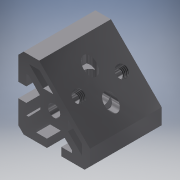
# Autodesk Inventor part: 21-035
Saved by Autodesk Inventor 2018 (Build 220105000, 105)
## iProperties
Created: 2004-10-14
Part Number: 21-035
Material: Aluminum-6061
Document SubType Name: Modeling
Designer: Autodesk, Inc.
Manufacturer: Standard
Standards Organization: Custom
Description: CORNER ELEMENT 1, 40
Catalog Web Link: http://www.parker.com/ead/cm1.asp?cmid=809
Vendor: PARKER IPS
Mass: 78.2567 g
Surface Area: 142.922 cm^2
Volume: 28.877 cm^3
Density: 2.71 g/cm^3
Appearance: Metal-AL-6061 (Polished)
CAGE: 1LJX3
Dept. ID: Product Design
Description #2: ---
Finish #1: ---
Finish #2: ---
Material ID: ---
Project Number: ---
Author: Autodesk, Inc.
Autodesk Inventor part; units mm, degrees
note: some values were not read from the file. Chosen so that the rebuilt part matches the saved one: direction of "Mounting Hole".
ref_plane "YZ Plane" through (0, 0, 0) normal (1, 0, 0) x (0, 1, 0)
ref_plane "XZ Plane" through (0, 0, 0) normal (0, 1, 0) x (-1, 0, 0)
sketch "Sketch1" plane through (0, 0, 0) normal (0, 0, 1) x (1, 0, 0)
  circle A0 centre (0, 0) radius 3.4
  line L0 (-8.3327, 20) -> (20, -8.3327)
  line L1 (20, -8.3327) -> (20, -17)
  line L2 (20, -17) -> (17, -20)
  line L3 (17, -20) -> (4, -20)
  line L4 (4, -20) -> (4, -15.5)
  line L5 (4, -15.5) -> (10, -15.5)
  line L6 (10, -15.5) -> (10, -14.177)
  line L7 (10, -14.177) -> (3.3741, -7.75)
  line L8 (3.3741, -7.75) -> (-3.3741, -7.75)
  line L9 (-3.3741, -7.75) -> (-10, -14.177)
  line L10 (-10, -14.177) -> (-10, -15.5)
  line L11 (-10, -15.5) -> (-4, -15.5)
  line L12 (-4, -15.5) -> (-4, -20)
  line L13 (-4, -20) -> (-17, -20)
  line L14 (-17, -20) -> (-20, -17)
  line L15 (-20, -17) -> (-20, -4)
  line L16 (-20, -4) -> (-15.5, -4)
  line L17 (-15.5, -4) -> (-15.5, -10)
  line L18 (-15.5, -10) -> (-14.177, -10)
  line L19 (-14.177, -10) -> (-7.75, -3.3741)
  line L20 (-7.75, -3.3741) -> (-7.75, 3.3741)
  line L21 (-7.75, 3.3741) -> (-14.177, 10)
  line L22 (-14.177, 10) -> (-15.5, 10)
  line L23 (-15.5, 10) -> (-15.5, 4)
  line L24 (-15.5, 4) -> (-20, 4)
  line L25 (-20, 4) -> (-20, 17)
  line L26 (-20, 17) -> (-17, 20)
  line L27 (-17, 20) -> (-8.3327, 20)
  line L28 (-6.1237, 7.75) -> (-13.8737, 15.5)
  line L29 (-13.8737, 15.5) -> (-8.2168, 15.5)
  line L30 (-8.2168, 15.5) -> (-0.4668, 7.75)
  line L31 (-0.4668, 7.75) -> (-6.1237, 7.75)
  line L32 (7.75, -6.1237) -> (15.5, -13.8737)
  line L33 (15.5, -13.8737) -> (15.5, -8.2168)
  line L34 (15.5, -8.2168) -> (7.75, -0.4668)
  line L35 (7.75, -0.4668) -> (7.75, -6.1237)
  constraints: 72 end point, 12 horizontal, 12 vertical, 1 centre point, 51 other
extrude "Extrusion1" add sketch "Sketch1" along normal mid plane 40
sketch "Sketch2" plane through (-3.3741, -7.75, 20) normal (0, -1, 0) x (1, 0, 0)
  line L0 (0, -40) -> (6.7482, -40) construction
  point P0 (3.3741, -20)
  point P1 (3.3741, -40)
  dimension "d2" = 20
  constraints: 1 midpoint, 1 vertical alignment
  measures "d2" distance from line of point (3.374, -20) L0
hole "Access Hole" at (0, -7.75, 0) direction (0, 1, 0) diameter 7 end through all
pattern_circular "Access Hole Pattern" count 2 over 90 about axis through (0, 0, -10) along (0, 0, -1) of "Access Hole"
mirror "Access Hole Mirrir" [suppressed]
ref_plane "Hole Terminal" through (-7.75, -3.3741, 20) normal (0.7071068, 0.7071068, 0) x (0.7071068, -0.7071068, 0)
sketch "Sketch3" plane through (20, -8.3327, -20) normal (0.7071068, 0.7071068, 0) x (-0.7071068, 0.7071068, 0)
  line L0 (40.0685, 40) -> (0, 40) construction
  point P0 (20.0343, 32)
  point P1 (20.0343, 40)
  dimension "d13" = 8
  constraints: 1 midpoint, 1 vertical alignment
  measures "d13" distance from line of point (20.034, 32) L0
hole "Mounting Hole" at (5.8336, 5.8336, 12) direction (-0.7071068, -0.7071068, 0) diameter 6.647 depth 16.1159 thread size "M8x1.25" class "6H" standard "ANSI Metric M Profile"
mirror "Mount Hole Mirror" about plane through (0, 0, 0) normal (0, 0, 1) of "Mounting Hole"
sketch "Sketch4" plane through (-20, -17, 20) normal (-0.7071068, -0.7071068, 0) x (-0.7071068, 0.7071068, 0)
  line L0 (-4.2426, 0) -> (0, 0) construction
  point P0 (-2.1213, 20)
  point P1 (-2.1213, 0)
  dimension "d21" = 20
  constraints: 1 midpoint, 1 vertical alignment
  measures "d21" distance from line of point (-2.121, 20) L0
hole "M8 Hole" [suppressed]
mirror "M8 Hole Mirror" [suppressed]
body "Solid1"
